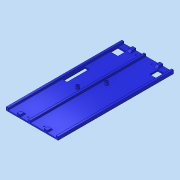
# Autodesk Inventor part: electronics_board_tray
Saved by Autodesk Inventor 2022 (Build 260153000, 153)
## iProperties
Created: 2020-11-04
Part Number: electronics_board_tray
Material: Generic
Document SubType Name: Modeling
Designer: nnico
Density: 1 g/cm^3
Appearance: Blue - Wall Paint - Glossy
Author: nnico
Autodesk Inventor part; units mm, degrees
ref_plane "YZ Plane" through (0, 0, 0) normal (1, 0, 0) x (0, 1, 0)
ref_plane "XZ Plane" through (0, 0, 0) normal (0, 1, 0) x (-1, 0, 0)
ref_plane "XY Plane" through (0, 0, 0) normal (0, 0, 1) x (1, 0, 0)
sketch "Sketch1" plane through (0, 0, 0) normal (0, 1, 0) x (-1, 0, 0)
  line L0 (65, -145) -> (-65, -145)
  line L1 (-65, -145) -> (-65, 145)
  line L2 (-65, 145) -> (65, 145)
  line L3 (65, 145) -> (65, -145)
  line L4 (65, 0) -> (-65, 0) construction
  line L5 (0, -145) -> (0, 145) construction
  point P0 (0, 0)
  point P1 (0, 0)
  dimension "d0" = 130
  dimension "d1" = 290
  constraints: 12 end point, 5 midpoint, 2 parallel, 1 coincident, 1 horizontal, 1 perpendicular
  measures "d0" distance of L1.end L2.end
  measures "d1" distance of L0.end L1.end
extrude "Extrusion1" add sketch "Sketch1" along normal blind 3
sketch "Sketch2" plane through (0, 0, 0) normal (0, -1, 0) x (1, 0, 0)
  line L0 (65, -145) -> (-65, -145) construction
  line L1 (0, -145) -> (0, 145) construction
  line L2 (-65, 145) -> (65, 145) construction
  line L3 (65, 145) -> (65, -145) construction
  line L4 (65, 0) -> (-65, 0) construction
  line L5 (-65, -145) -> (-65, 145) construction
  line L6 (-38, -145) -> (-30, -145)
  line L7 (-30, -145) -> (-30, -131)
  line L8 (-30, -131) -> (-38, -131)
  line L9 (-38, -131) -> (-38, -145)
  line L10 (38, -145) -> (30, -145)
  line L11 (30, -145) -> (30, -131)
  line L12 (30, -131) -> (38, -131)
  line L13 (38, -131) -> (38, -145)
  line L14 (-38, 145) -> (-30, 145)
  line L15 (-30, 145) -> (-30, 131)
  line L16 (-30, 131) -> (-38, 131)
  line L17 (-38, 131) -> (-38, 145)
  line L18 (30, 145) -> (30, 131)
  line L19 (38, 131) -> (38, 145)
  line L20 (30, 131) -> (38, 131)
  line L21 (38, 145) -> (30, 145)
  point P0 (0, 0)
  dimension "d4" = 8
  dimension "d5" = 14
  dimension "d6" = 30
  constraints: 36 end point, 12 symmetric about line, 4 midpoint, 2 parallel, 1 horizontal, 1 perpendicular, 1 point on line
  measures "d4" distance of L8.end L7.end
  measures "d5" distance of L7.end L6.end
  measures "d6" distance of L6.end L1.start
extrude "Extrusion2" add sketch "Sketch2" against normal blind 8
chamfer "Chamfer1" distance 5 angle 45 4 edges at (-34, 8, 131) (34, 8, 131) (-34, 8, -131) (34, 8, -131)
sketch "Sketch3" plane through (65, 0, -145) normal (0, 0, -1) x (-1, 0, 0)
  line L0 (65, 0) -> (65, 3) construction
  line L1 (35, 3) -> (95, 3) construction
  circle A0 centre (31, 4) radius 1.75
  line L2 (27, 8) -> (35, 8) projected
  line L3 (35, 3) -> (35, 8) projected
  circle A1 centre (99, 4) radius 1.75
  dimension "d12" = 3.5
  dimension "d13" = 4
  dimension "d14" = 4
  constraints: 2 centre point, 2 end point, 1 midpoint, 1 symmetric about line, 1 other
  measures "d12" diameter of A0
  measures "d13" distance from line of L2 A0.centre
  measures "d14" distance from line of L3 A0.centre
extrude "Extrusion3" cut sketch "Sketch3" against normal blind 6
sketch "Sketch4" plane through (-65, 0, 145) normal (0, 0, 1) x (1, 0, 0)
  circle A0 centre (99, 4) radius 1.75 projected
  circle A1 centre (31, 4) radius 1.75 projected
  point P0 (65, 0)
extrude "Extrusion4" cut sketch "Sketch4" against normal blind 6
sketch "Sketch5" plane through (0, 3, 0) normal (0, 1, 0) x (1, 0, 0)
  line L0 (-60, 130) -> (-40, 130)
  line L1 (-40, 130) -> (-40, 110)
  line L2 (-40, 110) -> (-60, 110)
  line L3 (-60, 110) -> (-60, 130)
  line L4 (-38, 145) -> (-65, 145) projected
  line L5 (-65, 145) -> (-65, -145) projected
  line L6 (-65, 145) -> (65, 145) construction
  line L7 (0, 145) -> (0, -145) construction
  line L8 (-30, -145) -> (30, -145) construction
  line L9 (60, 130) -> (40, 130)
  line L10 (40, 130) -> (40, 110)
  line L11 (40, 110) -> (60, 110)
  line L12 (60, 110) -> (60, 130)
  point P0 (0, 0)
  dimension "d19" = 20
  dimension "d20" = 20
  dimension "d21" = 15
  dimension "d22" = 5
  constraints: 18 end point, 4 symmetric about line, 2 midpoint, 2 parallel, 1 horizontal, 1 perpendicular
  measures "d19" distance of L1.end L2.end
  measures "d20" distance of L0.end L1.end
  measures "d21" distance from line of L4 L0.start
  measures "d22" distance between parallel lines of L5 L3
extrude "Extrusion5" cut sketch "Sketch5" against normal up to next
sketch "Sketch7" plane through (0, 3, 0) normal (0, 1, 0) x (1, 0, 0)
  line L0 (44, -14) -> (-25, -14) construction
  line L1 (-25, -14) -> (-25, 70) construction
  line L2 (-25, 70) -> (44, 70) construction
  line L3 (44, 70) -> (44, -14) construction
  line L4 (9.5, -14) -> (9.5, 70) construction
  line L5 (44, 28) -> (-25, 28) construction
  line L6 (-65, 145) -> (-65, -145) construction
  circle A0 centre (-21, -10) radius 4
  circle A1 centre (-21, -10) radius 2.25
  circle A2 centre (7, 35) radius 4
  circle A3 centre (7, 35) radius 2.25
  point P0 (0, 0)
  point P1 (40, 110)
  dimension "d39" = 69
  dimension "d40" = 84
  dimension "d41" = 40
  dimension "d42" = 40
  dimension "d43" = 8
  dimension "d44" = 4
  dimension "d45" = 4
  dimension "d46" = 4.5
  dimension "d49" = 8
  dimension "d50" = 49
  dimension "d51" = 32
  dimension "d52" = 4.5
  constraints: 12 end point, 4 centre point, 4 midpoint, 2 coincident, 2 parallel, 1 horizontal, 1 perpendicular
  measures "d39" distance of L0.start L0.end
  measures "d40" distance of L2.end L0.start
  measures "d41" distance from line of L6 L1.end
  measures "d42" distance from line of L2 point (40, 110)
  measures "d43" diameter of A0
  measures "d44" distance from line of L0 A0.centre
  measures "d45" distance from line of L1 A0.centre
  measures "d46" diameter of A1
  measures "d49" diameter of A2
  measures "d50" distance from line of L0 A2.centre
  measures "d51" distance from line of L1 A2.centre
  measures "d52" diameter of A3
extrude "Extrusion7" add sketch "Sketch7" along normal blind 6
sketch "Sketch8" plane through (0, 3, 0) normal (0, 1, 0) x (1, 0, 0)
  line L0 (-57.5, 45) -> (-47.5, 45)
  line L1 (-47.5, 45) -> (-47.5, -10)
  line L2 (-47.5, -10) -> (-57.5, -10)
  line L3 (-57.5, -10) -> (-57.5, 45)
  line L4 (-38, 145) -> (-65, 145) projected
  line L5 (-65, 145) -> (-65, -145) projected
  point P0 (0, 0)
  dimension "d53" = 10
  dimension "d54" = 100
  dimension "d55" = 55
  dimension "d56" = 7.5
  constraints: 8 end point, 2 parallel, 1 horizontal, 1 perpendicular
  measures "d53" distance of L1.end L2.end
  measures "d54" distance from line of L4 L0.start
  measures "d55" distance of L2.end L0.start
  measures "d56" distance from line of L5 L0.start
extrude "Extrusion8" cut sketch "Sketch8" against normal blind 6
sketch "Sketch9" plane through (0, 3, 0) normal (0, 1, 0) x (1, 0, 0)
  line L0 (65, -145) -> (-65, -145) construction
  line L1 (0, -145) -> (0, 145) construction
  line L2 (-65, 145) -> (65, 145) construction
  line L3 (65, 145) -> (65, -145) construction
  line L4 (65, 0) -> (-65, 0) construction
  line L5 (-65, -145) -> (-65, 145) construction
  line L6 (30, 145) -> (30, 131) construction
  line L7 (30, 135) -> (-30, 135) construction
  line L8 (-30, 131) -> (-30, 145) construction
  circle A0 centre (20, 135) radius 1.25
  circle A1 centre (-20, 135) radius 1.25
  circle A2 centre (20, -135) radius 1.25
  circle A3 centre (-20, -135) radius 1.25
  point P0 (0, 0)
  point P1 (30, 136)
  point P2 (-30, 136)
  dimension "d60" = 10
  dimension "d61" = 2.5
  dimension "d62" = 40
  constraints: 6 end point, 4 centre point, 4 midpoint, 3 point on line, 3 symmetric about line, 1 horizontal, 3 other
  measures "d60" distance between parallel lines of L2 L7
  measures "d61" diameter of A0
  measures "d62" diameter of A0.centre L1
extrude "Extrusion9" cut sketch "Sketch9" against normal blind 10
sketch "Sketch10" plane through (0, 3, 0) normal (0, 1, 0) x (1, 0, 0)
  line L0 (65, -145) -> (-65, -145) construction
  line L1 (0, -145) -> (0, 145) construction
  line L2 (-65, 145) -> (65, 145) construction
  line L3 (-65, -145) -> (-65, 145) projected
  line L4 (-65, -145) -> (-60, -145)
  line L5 (-60, -145) -> (-60, 145)
  line L6 (-60, 145) -> (-65, 145)
  line L7 (-65, 145) -> (-65, -145)
  line L8 (65, -145) -> (65, 145)
  line L9 (65, -145) -> (60, -145)
  line L10 (60, -145) -> (60, 145)
  line L11 (60, 145) -> (65, 145)
  line L12 (65, 145) -> (65, -145)
  point P0 (0, 0)
  dimension "d65" = 5
  constraints: 20 end point, 4 symmetric about line, 2 midpoint, 2 parallel, 1 horizontal, 1 perpendicular, 1 point on line
  measures "d65" distance of L6.end L5.end
extrude "Extrusion10" add sketch "Sketch10" along normal blind 5
sketch "Sketch11" plane through (0, 3, 0) normal (0, 1, 0) x (1, 0, 0)
  line L0 (65, -145) -> (-65, -145) projected
  line L1 (-65, 145) -> (65, 145) projected
  line L2 (-4.5, -145) -> (-9.5, -145)
  line L3 (-9.5, -145) -> (-9.5, 145)
  line L4 (-9.5, 145) -> (-4.5, 145)
  line L5 (-4.5, 145) -> (-4.5, -145)
  circle A0 centre (-21, -10) radius 4 projected
  point P0 (0, 0)
  dimension "d68" = 5
  dimension "d69" = 11.5
  constraints: 8 end point, 2 parallel, 2 point on line, 1 horizontal, 1 perpendicular
  measures "d68" distance of L2.start L2.end
  measures "d69" distance from line of A0.centre L3
extrude "Extrusion11" add sketch "Sketch11" along normal blind 5 contours L0 L3 L1 L5
body "Solid1"
